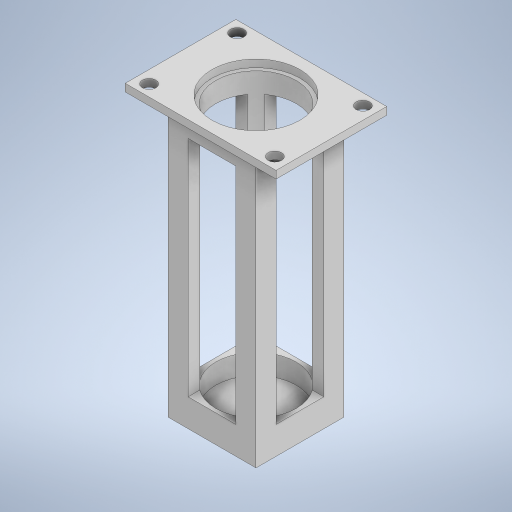
# Autodesk Inventor part: port tube v01
Saved by Autodesk Inventor 2023.5 (Build 275446000, 446)
## iProperties
Created: 2024-09-06
Part Number: port tube v01
Material: Generic
Document SubType Name: Modeling
Designer: Akramilab
Density: 1 g/cm^3
Appearance: Default
Author: Akramilab
Autodesk Inventor part; units mm, degrees
ref_plane "YZ Plane" through (0, 0, 0) normal (1, 0, 0) x (0, 1, 0)
ref_plane "XZ Plane" through (0, 0, 0) normal (0, 1, 0) x (-1, 0, 0)
ref_plane "XY Plane" through (0, 0, 0) normal (0, 0, 1) x (1, 0, 0)
sketch "Sketch1" plane through (0, 0, 0) normal (0, 1, 0) x (-1, 0, 0)
  line L0 (17.5, 17.5) -> (-17.5, 17.5)
  line L1 (-17.5, 17.5) -> (-17.5, -17.5)
  line L2 (-17.5, -17.5) -> (17.5, -17.5)
  line L3 (17.5, -17.5) -> (17.5, 17.5)
  line L4 (17.5, 17.5) -> (-17.5, -17.5) construction
  line L5 (-17.5, 17.5) -> (17.5, -17.5) construction
  circle A0 centre (0, 0) radius 16
  dimension "d0" = 35
  dimension "d1" = 35
  dimension "d2" = 32
  constraints: 12 end point, 2 midpoint, 2 parallel, 1 centre point, 1 coincident, 1 horizontal, 1 perpendicular
  measures "d0" distance of L0.end L1.end
  measures "d1" distance of L1.end L2.end
  measures "d2" diameter of A0
extrude "Extrusion1" add sketch "Sketch1" along normal blind 105
sketch "Sketch2" plane through (17.5, 0, 17.5) normal (1, 0, 0) x (0, 0, -1)
  line L0 (27, 8) -> (8, 8)
  line L1 (8, 8) -> (8, 97)
  line L2 (8, 97) -> (27, 97)
  line L3 (27, 97) -> (27, 8)
  line L4 (0, 0) -> (35, 0) projected
  line L5 (0, 0) -> (0, 105) projected
  line L6 (35, 0) -> (35, 105) projected
  line L7 (0, 105) -> (35, 105) projected
  point P0 (17.5, 0)
  dimension "d5" = 8
  dimension "d6" = 8
  dimension "d7" = 8
  dimension "d8" = 8
  constraints: 8 end point, 2 parallel, 1 horizontal, 1 perpendicular
  measures "d5" distance between parallel lines of L0 L4
  measures "d6" distance between parallel lines of L5 L1
  measures "d7" distance between parallel lines of L3 L6
  measures "d8" distance between parallel lines of L2 L7
extrude "Extrusion2" cut sketch "Sketch2" against normal through all contours L0 L1 L2 L3
sketch "Sketch3" plane through (17.5, 0, -17.5) normal (0, 0, -1) x (-1, 0, 0)
  line L0 (8, 97) -> (27, 97)
  line L1 (27, 97) -> (27, 8)
  line L2 (27, 8) -> (8, 8)
  line L3 (8, 8) -> (8, 97)
  line L4 (0, 0) -> (0, 105) projected
  line L5 (35, 0) -> (35, 105) projected
  line L6 (0, 105) -> (35, 105) projected
  line L7 (0, 0) -> (35, 0) projected
  point P0 (17.5, 0)
  dimension "d11" = 8
  dimension "d12" = 8
  dimension "d13" = 8
  dimension "d14" = 8
  constraints: 8 end point, 2 parallel, 1 horizontal, 1 perpendicular
  measures "d11" distance between parallel lines of L4 L3
  measures "d12" distance between parallel lines of L1 L5
  measures "d13" distance between parallel lines of L0 L6
  measures "d14" distance between parallel lines of L7 L2
extrude "Extrusion3" cut sketch "Sketch3" against normal through all contours L0 L1 L2 L3
sketch "Sketch4" plane through (0, 0, 0) normal (0, -1, 0) x (1, 0, 0)
  line L0 (17.5, 17.5) -> (17.5, -17.5) projected
  line L1 (-17.5, 17.5) -> (17.5, 17.5)
  line L2 (17.5, 17.5) -> (17.5, -17.5)
  line L3 (17.5, -17.5) -> (-17.5, -17.5)
  line L4 (-17.5, -17.5) -> (-17.5, 17.5)
  line L5 (-17.5, 17.5) -> (17.5, -17.5) construction
  line L6 (17.5, 17.5) -> (-17.5, -17.5) construction
  point P0 (0, 0)
  constraints: 12 end point, 2 midpoint, 2 parallel, 1 horizontal, 1 perpendicular
extrude "Extrusion4" add sketch "Sketch4" along normal blind 3
sketch "Sketch5" plane through (0, 105, 0) normal (0, 1, 0) x (1, 0, 0)
  line L0 (30, 22) -> (-30, 22)
  line L1 (-30, 22) -> (-30, -22)
  line L2 (-30, -22) -> (30, -22)
  line L3 (30, -22) -> (30, 22)
  line L4 (30, 22) -> (-30, -22) construction
  line L5 (-30, 22) -> (30, -22) construction
  circle A0 centre (0, 0) radius 17.5
  circle A1 centre (25, -17.5) radius 2.7
  circle A2 centre (25, 17.5) radius 2.7
  circle A3 centre (-25, 17.5) radius 2.7
  circle A4 centre (-25, -17.5) radius 2.7
  dimension "d19" = 60
  dimension "d20" = 44
  dimension "d21" = 35
  dimension "d22" = 5.4
  dimension "d23" = 4.5
  dimension "d24" = 5
  dimension "d25" = 5.4
  dimension "d26" = 4.5
  dimension "d27" = 5
  dimension "d28" = 4.5
  dimension "d29" = 5
  dimension "d30" = 5.4
  dimension "d31" = 5.4
  dimension "d32" = 4.5
  dimension "d33" = 5
  constraints: 12 end point, 5 centre point, 2 midpoint, 2 parallel, 1 coincident, 1 horizontal, 1 perpendicular
  measures "d19" distance of L2.end L1.end
  measures "d20" distance of L1.end L0.end
  measures "d21" diameter of A0
  measures "d22" diameter of A1
  measures "d23" distance from line of L2 A1.centre
  measures "d24" distance from line of L3 A1.centre
  measures "d25" diameter of A2
  measures "d26" distance from line of A2.centre L0
  measures "d27" distance from line of L3 A2.centre
  measures "d28" distance from line of A3.centre L0
  measures "d29" distance from line of A3.centre L1
  measures "d30" diameter of A4
  measures "d31" diameter of A3
  measures "d32" distance from line of A4.centre L2
  measures "d33" distance from line of L1 A4.centre
extrude "Extrusion5" add sketch "Sketch5" along normal blind 3
equation "\"d0\" = d1"
equation "\"d6\" = d5"
equation "\"d7\" = d6"
equation "\"d8\" = d5"
equation "\"d12\" = d11"
equation "\"d13\" = d11"
equation "\"d14\" = d11"
equation "\"d25\" = d22"
equation "\"d26\" = d23"
equation "\"d27\" = d24"
equation "\"d28\" = d32"
equation "\"d29\" = d24"
equation "\"d30\" = d22"
equation "\"d31\" = d22"
equation "\"d32\" = d23"
equation "\"d33\" = d24"
body "Solid1"
